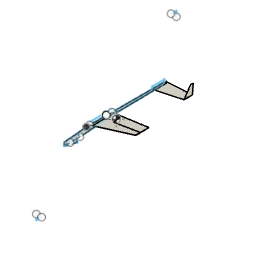
WingSample v3 (Autodesk Fusion 360 design; units mm, degrees)
Autodesk Fusion 360 part; units mm, degrees
note: some values were not read from the file. Set by a fixed rule: which sketch regions a step uses.
sketch "スケッチ4" plane through (0, 0, 0) normal (1, 0, 0) x (0, 1, 0)
  line L0 (-131.99, -95) -> (-131.99, -105)
  line L1 (-131.99, -105) -> (-121.99, -105)
  line L2 (131.99, 95) -> (131.99, 105)
  line L3 (131.99, 105) -> (121.99, 105)
  line L4 (0, -10) -> (0, 0)
  line L5 (-1.82, -5) -> (-1.82, 0)
  line L6 (-74.01, 0) -> (111.99, 0)
  line L7 (-26.4634, 85) -> (-1.4634, 85)
  line L8 (-31.29, 0) -> (-26.4634, 85)
  line L9 (-1.4634, 85) -> (10.71, 0)
  line L10 (98.9878, 47.61) -> (114.7578, 47.61)
  line L11 (116.4027, 66.31) -> (114.7578, 47.61)
  line L12 (85.99, 0) -> (98.9878, 47.61)
  line L13 (98.9878, 47.61) -> (111.4027, 66.31)
  line L14 (114.7578, 47.61) -> (111.99, 0)
  line L15 (111.4027, 66.31) -> (116.4027, 66.31)
sketch "スケッチ5" plane through (0, 0, 0) normal (1, 0, 0) x (0, 1, 0)
  line L0 (-131.99, -95) -> (-131.99, -105)
  line L1 (-31.29, 0) -> (10.71, 0)
  line L2 (98.9878, 47.61) -> (111.4027, 66.31)
  line L3 (98.9878, 47.61) -> (114.7578, 47.61)
  line L4 (-26.4634, 85) -> (-1.4634, 85)
  line L5 (114.7578, 47.61) -> (111.99, 0)
  line L6 (111.4027, 66.31) -> (116.4027, 66.31)
  line L7 (116.4027, 66.31) -> (114.7578, 47.61)
  line L8 (131.99, 105) -> (121.99, 105)
  line L9 (-31.29, 0) -> (-26.4634, 85)
  line L10 (85.99, 0) -> (98.9878, 47.61)
  line L11 (-131.99, -105) -> (-121.99, -105)
  line L12 (-1.4634, 85) -> (10.71, 0)
  line L13 (131.99, 95) -> (131.99, 105)
  line L14 (-17.3015, 85) -> (-10.4991, 25.5069)
  line L15 (-10.4991, 25.5069) -> (7.7428, 20.7181)
  line L16 (111.99, 0) -> (111.99, -5)
  line L17 (0, 0) -> (0, 0.97)
  line L18 (85.99, 0) -> (111.99, 0) construction
  line L19 (85.99, 0) -> (111.99, 0)
  dimension "d1" = 5
  constraint coincident L4 L14.start
  constraint coincident L12 L15.end
  constraint perpendicular L1 L16
  constraint perpendicular L1 L17
  constraint horizontal L18
  constraint perpendicular L16 L19
  measures "d1" distance of L5.end L16.end
sketch "スケッチ7" plane through (0, 0, 0) normal (1, 0, 0) x (0, 1, 0)
  line L0 (-37.4436, 0) -> (85.99, 0)
  line L1 (0, 0) -> (0, 0.97)
  line L2 (-37.4436, 0) -> (-79.1405, -4.0764)
  line L3 (85.99, 0) -> (109.7552, 0.2074)
  line L4 (-131.99, -105) -> (-121.99, -105)
  line L5 (131.99, 95) -> (131.99, 105)
  line L6 (131.99, 105) -> (121.99, 105)
  line L7 (-79.1405, -4.0764) -> (-79.1405, -10.2977)
  line L8 (-131.99, -95) -> (-131.99, -105)
  line L9 (85.99, 0) -> (86.6072, 4.0055)
  line L10 (109.7203, 4.2072) -> (86.6072, 4.0055)
  line L11 (-31.29, 0) -> (-31.0061, 5)
  line L12 (0, 0) -> (0, 0.97)
  line L13 (9.9939, 5) -> (10.71, 0)
  line L14 (9.9939, 5) -> (-31.0061, 5)
  line L15 (-79.1405, -10.2977) -> (-54.0753, -16.752)
  line L16 (-54.0753, -16.752) -> (-57.5465, -10.0488)
  line L17 (-37.4436, 0) -> (-28.9612, -8.5322)
  line L18 (17.8102, 0) -> (21.81, -4.9375)
  line L19 (105.9441, -3.6515) -> (13.5108, -5.0644)
  line L20 (-57.5465, -10.0488) -> (-79.1405, -10.2977)
  line L21 (-57.5465, -10.0488) -> (-68.3435, -10.1732)
  line L22 (-57.5465, -10.0488) -> (-45.8903, -9.9145)
  line L23 (-45.8903, -9.9145) -> (13.5108, -5.0644)
  line L24 (109.7203, 4.2072) -> (109.7552, 0.2074)
  line L25 (109.7552, 0.2074) -> (105.9441, -3.6515)
  line L26 (-54.6157, -1.6788) -> (-49.6153, -9.9817)
  point P0 (-37.4436, 0)
  constraint perpendicular L0 L1
  constraint vertical L7
  constraint parallel L3 L10
  constraint coincident L2 P0
  constraint coincident L0 L18.start
  constraint coincident L19 L18.end
  constraint coincident P0 L0.start
  constraint parallel L20 L21
  constraint parallel L21 L22
  constraint coincident L23 L17.end
  constraint perpendicular L3 L24
  constraint coincident L2 L26.start
extrude "押し出し1" add sketch "スケッチ5" along normal blind 0.2 contours L1 L4 L9 L12 L14 L15 | L4 L12 L14 L15 makes body 1
extrude "押し出し2" add sketch "スケッチ5" along normal blind 0.2 separate body contours L1 L4 L9 L12 L14 L15 makes body 2
extrude "押し出し3" add sketch "スケッチ5" along normal blind 0.2 separate body contours L3 L5 L10 L19 makes body 3
extrude "押し出し4" add sketch "スケッチ5" along normal blind 0.2 separate body contours L2 L3 L6 L7 makes body 4
move_body "移動1" bodies 4 to x (0, 0, 1) y (0, 1, 0) z (-1, 0, 0) at (47.81, 0, 47.41)
combine "結合1" operation add target body 3 tool bodies 4
move_body "移動2" bodies 1 to x (1, 0, 0) y (0, 1, 0) z (0, 0, 1) at (-0.2, 0, 0)
move_body "移動3" bodies 3 to x (0, 0, -1) y (0, 1, 0) z (1, 0, 0) at (0, 0, 0)
move_body "移動4" bodies 1 2 to x (0.258819, 0, -0.965926) y (0, 1, 0) z (0.965926, 0, 0.258819) at (-0.1482, 0, -0.1932)
extrude "押し出し5" add sketch "スケッチ7" along normal blind 0.2 separate body contours L0 L17 L18 L19 L23 | L2 L7 L20 L21 L22 L26 | L15 L16 L20 L21 | L0 L3 L18 L19 L25 makes body 5 at (0, -63.7676, -5.268) makes body 6 at (0, -17.6314, -4.5322)
extrude "押し出し6" add sketch "スケッチ7" along normal blind 0.2 separate body contours L0 L17 L18 L19 L23 | L2 L7 L20 L21 L22 L26 | L15 L16 L20 L21 | L0 L3 L18 L19 L25 makes body 7 at (0, -63.7676, -5.268) makes body 8 at (0, -17.6314, -4.5322)
extrude "押し出し7" add sketch "スケッチ7" along normal blind 0.2 separate body contours L3 L9 L10 L24 makes body 9
move_body "移動5" bodies 9 to x (0, 0.008727, -0.999962) y (-0.008727, 0.999924, 0.008726) z (0.999962, 0.008726, 0.000076) at (0.7504, 0.0065, -0.7504)
combine "結合2" operation add target body 7 tool bodies 9 makes body 10 at (1.3333, 94.1291, 0.071)
extrude "押し出し8" add sketch "スケッチ7" along normal blind 0.2 separate body contours L0 L17 L18 L19 L23 | L2 L7 L20 L21 L22 L26 makes body 11 at (0, -17.6314, -4.5322) makes body 12 at (0, -61.1287, -7.3113)
extrude "押し出し9" add sketch "スケッチ7" along normal blind 0.2 separate body contours L0 L11 L13 L14 makes body 13
move_body "移動6" bodies 13 to x (0.258819, 0, -0.965926) y (0, 1, 0) z (0.965926, 0, 0.258819) at (0, 0, 0)
combine "結合3" [no effect]
extrude "押し出し10" add sketch "スケッチ7" along normal blind 0.2 separate body contours L2 L7 L20 L21 L22 L26 makes body 14
extrude "押し出し11" add sketch "スケッチ7" along normal blind 0.1 separate body contours L2 L7 L20 L21 L22 L26 makes body 15
extrude "押し出し12" add sketch "スケッチ7" along normal blind 0.2 contours L2 L17 L22 L23 L26 bodies 5 6
extrude "押し出し13" add sketch "スケッチ7" along normal blind 0.2 contours L2 L17 L22 L23 L26 bodies 7 10 8
combine "結合4" operation add target body 7 tool bodies 10
extrude "押し出し14" add sketch "スケッチ7" along normal blind 0.2 contours L2 L17 L22 L23 L26 bodies 11 13 12
combine "結合5" operation add target body 11 tool bodies 13
move_face "面を移動1" by (0.1, 0, 0) 1 faces at (0.1, -67.3666, -5.3095) on bodies 15
extrude "押し出し15" add sketch "スケッチ7" along normal blind 0.2 contours L2 L17 L22 L23 L26 bodies 14
named bodies: "W1", "W2", "T1", "T2", "B1", "B2", "B4", "B2 (1)", "B3", "B3 (1)", "B5"
